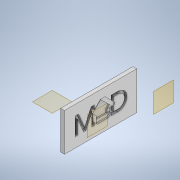
# Autodesk Inventor part: pare_choc_demo_2
Saved by Autodesk Inventor 2020.4 (Build 244396000, 396)
## iProperties
Created: 2021-07-13
Part Number: pare_choc_demo_2
Material: Generic
Document SubType Name: Modeling
Designer: Antonin Betaille
Density: 1 g/cm^3
Appearance: Default
Author: Antonin Betaille
Autodesk Inventor part; units mm, degrees
ref_plane "YZ Plane" through (0, 0, 0) normal (1, 0, 0) x (0, 1, 0)
ref_plane "XZ Plane" through (0, 0, 0) normal (0, 1, 0) x (-1, 0, 0)
ref_plane "XY Plane" through (0, 0, 0) normal (0, 0, 1) x (1, 0, 0)
ref_plane "Work Plane7" through (0, 4, 0) normal (0, 1, 0) x (1, 0, 0)
sketch "Sketch3" plane through (0, 4, 0) normal (0, 1, 0) x (1, 0, 0)
  line L0 (53, -39.5369) -> (53, 40.4631)
  line L1 (48.8, 40.4631) -> (48.8, -39.5369)
  line L2 (53, -38) -> (53, 38) projected
  line L3 (53, -39.5369) -> (48.8, -39.5369)
  line L4 (48.8, 40.4631) -> (53, 40.4631)
  line L5 (-0.4144, 0.0131) -> (73.2599, 0.0131)
  dimension "d42" = 80
  dimension "d43" = 4.2
  dimension "d468" = 80.9001
  constraints: 10 end point, 3 horizontal, 2 parallel, 1 collinear
  measures "d42" distance of L0.start L0.end
  measures "d43" distance between parallel lines of L1 L0
  measures "d468" diameter of L4 L5
extrude "Extrusion2" add sketch "Sketch3" along normal blind 38 and the other way blind 4
ref_plane "Work Plane5" through (53, 0, -70) normal (1, 0, 0) x (0, 0, -1)
sketch "Sketch4" plane through (53, 0, -70) normal (1, 0, 0) x (0, 0, -1)
  line L0 (-97.7445, 11.15) -> (-95.0445, 11.15)
  line L1 (-95.0445, 26.29) -> (-88.5241, 11.15)
  line L2 (-88.5241, 11.15) -> (-85.7871, 11.15)
  line L3 (-85.7871, 11.15) -> (-79.2667, 26.29)
  line L4 (-79.2667, 26.29) -> (-79.2667, 22.5482)
  line L5 (-79.2667, 26.29) -> (-79.2667, 11.15)
  line L6 (-76.5667, 30.85) -> (-79.0667, 30.85)
  arc A0 (-93.5854, 29.7482) -> (-95.2445, 30.85) centre (-95.2445, 29.05) ccw
  arc A1 (-79.0667, 30.85) -> (-80.7258, 29.7482) centre (-79.0667, 29.05) ccw
  line L7 (-93.5854, 29.7482) -> (-87.1558, 14.47)
  line L8 (-80.7258, 29.7482) -> (-87.1558, 14.47)
  line L9 (-97.7445, 11.15) -> (-97.7445, 30.85)
  line L10 (-97.7445, 30.85) -> (-95.2445, 30.85)
  line L11 (-76.5667, 30.85) -> (-76.5667, 11.15)
  line L12 (-79.2667, 11.15) -> (-76.5667, 11.15)
  line L13 (-95.0445, 11.15) -> (-95.0445, 26.29)
  point P0 (-70, 0)
  dimension "d117" = 1.8
  dimension "d118" = 1.8
  dimension "d119" = 2.5
  dimension "d120" = 2.5
  dimension "d124" = 19.7
  dimension "d136" = 1.6591
  dimension "d137" = 1.6591
  dimension "d143" = 15.14
  dimension "d144" = 15.14
  dimension "d147" = 3.32
  dimension "d161" = 2.7
  dimension "d180" = 2.7
  dimension "d185" = 23.3
  dimension "d186" = 23.3
  constraints: 28 end point, 6 point on line, 4 point on circle, 4 tangent, 3 horizontal, 3 vertical, 2 centre point, 1 parallel, 1 perpendicular
  measures "d117" radius of A0
  measures "d118" radius of A1
  measures "d119" distance of L9.end L10.end
  measures "d120" distance of L6.start L6.end
  measures "d124" distance between parallel lines of L10 L2
  measures "d136" horizontal distance of L7.start L10.end
  measures "d137" horizontal distance of L6.end L8.start
  measures "d143" distance from line of L0 L1.start
  measures "d144" distance from line of L12 L3.end
  measures "d147" distance from line of L2 L7.end
  measures "d161" distance of L5.end L11.end
  measures "d180" distance of L0.start L0.end
  measures "d185" angle of L13 L1
  measures "d186" angle of L3 L5
extrude "Extrusion3" cut sketch "Sketch4" against normal blind 2.8
ref_plane "Work Plane4" through (53, 0, -70) normal (1, 0, 0) x (0, 0, -1)
sketch "Sketch5" plane through (53, 0, -70) normal (1, 0, 0) x (0, 0, -1)
  line L0 (-79.0667, 30.85) -> (-76.5667, 30.85) projected
  line L1 (-57.8532, 30.85) -> (-50.2732, 30.85)
  line L2 (-76.5667, 11.15) -> (-79.2667, 11.15) projected
  line L3 (-50.2732, 11.15) -> (-57.8532, 11.15)
  line L4 (-57.8532, 30.85) -> (-57.8532, 11.15)
  line L5 (-55.1532, 28.15) -> (-50.2732, 28.15)
  line L6 (-55.1532, 28.15) -> (-55.1532, 13.85)
  line L7 (-55.1532, 13.85) -> (-50.2732, 13.85)
  arc A0 (-50.2732, 11.15) -> (-50.2732, 30.85) centre (-50.2732, 21) ccw
  arc A1 (-50.2732, 13.85) -> (-50.2732, 28.15) centre (-50.2732, 21) ccw
  line L8 (-76.5667, 30.85) -> (-76.5667, 11.15) projected
  point P0 (-70, 0)
  dimension "d259" = 2.7
  dimension "d262" = 2.7
  dimension "d263" = 2.7
  dimension "d267" = 18.7136
  dimension "d269" = 4.88
  dimension "d274" = 7.15
  dimension "d276" = 4.88
  constraints: 12 end point, 4 point on circle, 2 centre point, 2 collinear, 2 tangent, 1 coincident, 1 horizontal, 1 parallel, 1 perpendicular, 1 vertical
  measures "d259" distance between parallel lines of L6 L4
  measures "d262" radial gap between concentric circles of A0 A1
  measures "d263" distance between parallel lines of L5 L1
  measures "d267" distance between parallel lines of L4 L8
  measures "d269" distance of L6.end L7.end
  measures "d274" distance from line of L7 A1.centre
  measures "d276" distance from line of L6 A0.centre
extrude "Extrusion4" cut sketch "Sketch5" against normal blind 2.8
ref_plane "Work Plane3" through (53, 0, -70) normal (1, 0, 0) x (0, 0, -1)
sketch "Sketch6" plane through (53, 0, -70) normal (1, 0, 0) x (0, 0, -1)
  line L0 (-80.7188, 21.8815) -> (-69.814, 32.7863)
  line L1 (-69.814, 32.7863) -> (-64.5814, 32.7863)
  line L2 (-79.2667, 11.15) -> (-79.2667, 26.29) projected
  line L3 (-64.5814, 32.7863) -> (-53.6767, 21.8815)
  line L4 (-53.6767, 21.8815) -> (-55.3092, 18.2815)
  line L5 (-55.3092, 18.2815) -> (-57.3477, 18.2815)
  line L6 (-57.8532, 11.15) -> (-57.8532, 30.85) projected
  line L7 (-57.3477, 18.2815) -> (-57.3477, 14.3863)
  line L8 (-57.3477, 14.3863) -> (-60.9477, 10.7863)
  line L9 (-60.9477, 10.7863) -> (-73.4477, 10.7863)
  line L10 (-73.4477, 10.7863) -> (-77.0477, 14.3863)
  line L11 (-77.0477, 14.3863) -> (-77.0477, 18.2815)
  line L12 (-77.0477, 18.2815) -> (-79.0862, 18.2815)
  line L13 (-79.0862, 18.2815) -> (-80.7188, 21.8815)
  line L14 (-73.4477, 14.3863) -> (-73.4477, 18.2815)
  line L15 (-73.4477, 18.2815) -> (-76.267, 21.1008)
  line L16 (-76.267, 21.1008) -> (-67.1977, 30.17)
  line L17 (-67.1977, 30.17) -> (-58.1285, 21.1008)
  line L18 (-58.1285, 21.1008) -> (-60.9477, 18.2815)
  line L19 (-60.9477, 18.2815) -> (-60.9477, 14.3863)
  line L20 (-60.9477, 14.3863) -> (-73.4477, 14.3863)
  line L21 (-57.8532, 11.15) -> (-57.8532, 30.85) projected
  line L22 (-76.5667, 30.85) -> (-76.5667, 11.15) projected
  line L23 (-140, 0) -> (0, 0) projected
  line L24 (-69.814, 32.7863) -> (-55.3092, 18.2815)
  line L25 (-79.0862, 18.2815) -> (-64.5814, 32.7863)
  line L26 (-76.267, 21.1008) -> (-58.1285, 21.1008)
  line L27 (-80.7188, 21.8815) -> (-53.6767, 21.8815)
  line L28 (-77.0477, 18.2815) -> (-77.0477, 21.8815)
  line L29 (-76.267, 21.1008) -> (-77.0477, 21.8815)
  line L30 (-73.4477, 10.7863) -> (-73.4477, 14.3863)
  line L31 (-60.9477, 10.7863) -> (-60.9477, 14.3863)
  line L32 (-57.3477, 18.2815) -> (-60.9477, 18.2815)
  line L33 (-60.9477, 14.3863) -> (-57.3477, 14.3863)
  point P0 (-70, 0)
  point P1 (-76.5667, 13.9053)
  point P2 (-76.5667, 26.0336)
  point P3 (-79.2667, 23.3336)
  point P4 (-79.2667, 18.6795)
  point P5 (-57.8532, 26.0581)
  point P6 (-57.8532, 13.8809)
  point P7 (-57.8532, 14.3863)
  dimension "d311" = 3.7
  dimension "d316" = 3.7
  dimension "d366" = 12.5
  dimension "d389" = 3.6
  dimension "d390" = 3.6
  dimension "d406" = 2.0385
  dimension "d434" = 3.119
  dimension "d442" = 10.7863
  dimension "d447" = 3.6
  dimension "d448" = 22
  constraints: 58 end point, 10 parallel, 10 perpendicular, 10 point on line, 2 collinear, 1 horizontal
  measures "d311" distance between parallel lines of L16 L0
  measures "d316" distance between parallel lines of L17 L3
  measures "d366" distance of L8.end L9.end
  measures "d389" horizontal distance of L9.end L10.end
  measures "d390" distance from line of L9 L7.end
  measures "d406" distance of L11.end L12.end
  measures "d434" distance from line of L22 L9.end
  measures "d442" distance between parallel lines of L23 L9
  measures "d447" distance between parallel lines of L9 L20
  measures "d448" distance between parallel lines of L9 L1
extrude "Extrusion6" cut sketch "Sketch6" against normal blind 2.8 contours L27 L2 L13 | L0 L2 L27 | L0 L24 L16 L27 L22 | L1 L25 L24 | L27 L16 L29 L22 | L29 L25 L22 | L3 L6 L27 L17 L25 | L25 L15 L14 L30 L10 L22 | L3 L27 L6 | L27 L6 L24 L17 | L24 L6 L32 L18 | L4 L24 L6 L27 | L30 L20 L31 L9 | L32 L6 L33 L19 | L24 L5 L32 L6 | L31 L33 L6 L8 | L32 L7 L33 L6 | L6 L33 L8
ref_plane "Work Plane6" through (53, 14.3863, 3.4477) normal (1, 0, 0) x (0, 0, -1)
sketch "Sketch8" plane through (53, 14.3863, 3.4477) normal (1, 0, 0) x (0, 0, -1)
  line L0 (6.25, 15.7837) -> (-2.8192, 6.7145) projected
  line L1 (-2.8192, 6.7145) -> (6.25, 15.7837)
  line L2 (6.25, 15.7837) -> (15.3193, 6.7145)
  line L3 (12.5, 0) -> (12.5, 3.8952) projected
  line L4 (15.3193, 6.7145) -> (12.5, 3.8952)
  line L5 (12.5, 3.8952) -> (12.5, 0)
  line L6 (12.5, 0) -> (0, 0)
  line L7 (0, 0) -> (0, 3.8952)
  line L8 (-2.8192, 6.7145) -> (0, 3.8952) projected
  line L9 (0, 3.8952) -> (-2.8192, 6.7145)
  point P0 (3.4477, -14.3863)
  constraints: 14 end point, 4 perpendicular, 3 collinear
extrude "Extrusion10" cut sketch "Sketch8" against normal blind 2.8
extrude "Extrusion13" add sketch "Sketch6" along normal blind 1.8 from surface at -2.8 contours L29 L22 L25 L28 | L1 L25 L24 | L28 L25 L22 L10 L11 | L29 L25 L22 | L3 L6 L27 L17 L25 | L25 L15 L14 L30 L10 L22 | L3 L27 L6 | L27 L6 L24 L17 | L4 L24 L6 L27
extrude "Extrusion14" add sketch "Sketch6" along normal blind 1.2 from surface at -2.8 contours L27 L2 L13 | L2 L27 L28 L25 L13 | L25 L28 L12 | L24 L6 L32 L18 | L30 L20 L31 L9 | L24 L5 L32 L6 | L31 L33 L6 L8
extrude "Extrusion15" add sketch "Sketch6" along normal blind 0.6 from surface at -2.8 contours L0 L2 L27 | L0 L22 L27 L2 | L0 L24 L16 L27 L22 | L27 L22 L29 | L27 L16 L29 L22 | L32 L6 L33 L19 | L32 L7 L33 L6
body "Solid1"
